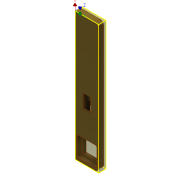
# Autodesk Inventor part: Hilla
Saved by Autodesk Inventor 2018 (Build 220112000, 112)
## iProperties
Created: 2019-09-21
Part Number: Hilla
Material: Lauan, Meranti
Document SubType Name: Modeling
Designer: ottar
Density: 0.416 g/cm^3
Appearance: Mahogany - Solid Stained Dark Medium Gloss
Author: ottar
Autodesk Inventor part; units mm, degrees
ref_plane "YZ Plane" through (0, 0, 0) normal (1, 0, 0) x (0, 1, 0)
ref_plane "XZ Plane" through (0, 0, 0) normal (0, 1, 0) x (-1, 0, 0)
sketch "Sketch1" plane through (0, 0, 0) normal (0, 1, 0) x (-1, 0, 0)
  line L0 (0, 0) -> (90, 0)
  line L1 (90, 0) -> (90, -500)
  line L2 (90, -500) -> (0, -500)
  line L3 (0, -500) -> (0, 0)
  dimension "d0" = 90
  dimension "d1" = 500
  constraints: 8 end point, 2 parallel, 1 horizontal, 1 perpendicular
  measures "d0" distance of L1.end L2.end
  measures "d1" distance of L0.end L1.end
extrude "Extrusion1" add sketch "Sketch1" along normal blind 25
sketch "Sketch6" plane through (0, 25, 0) normal (0, 1, 0) x (1, 0, 0)
  line L0 (-57.55, 311.9) -> (-32.45, 311.9)
  line L1 (-32.45, 311.9) -> (-32.45, 400)
  line L2 (-32.45, 400) -> (-57.55, 400)
  line L3 (-57.55, 400) -> (-57.55, 311.9)
  line L4 (-90, 500) -> (-90, 0) projected
  line L5 (0, 500) -> (-90, 500) projected
  point P0 (0, 0)
  dimension "d36" = 25.1
  dimension "d37" = 88.1
  dimension "d38" = 32.45
  dimension "d39" = 100
  constraints: 8 end point, 2 parallel, 1 horizontal, 1 perpendicular
  measures "d36" distance of L2.end L1.end
  measures "d37" distance of L0.end L1.end
  measures "d38" distance between parallel lines of L4 L3
  measures "d39" distance between parallel lines of L5 L2
extrude "Extrusion6" cut sketch "Sketch6" against normal blind 20
sketch "Sketch7" plane through (-32.45, 25, -311.9) normal (0, 0, -1) x (-1, 0, 0)
  line L0 (0, 0) -> (25.1, 0) projected
  line L1 (0, 0) -> (0, -20) projected
  line L2 (0, -20) -> (25.1, -20) projected
  line L3 (25.1, 0) -> (25.1, -20) projected
  line L4 (0, -4) -> (25.1, -4)
  line L5 (25.1, -4) -> (25.1, -23)
  line L6 (0, -4) -> (0, -23)
  line L7 (25.1, -23) -> (0, -23)
  point P0 (-32.45, -25)
  dimension "d42" = 16
  dimension "d43" = 19
  dimension "d44" = 19
  constraints: 8 end point, 2 vertical, 1 horizontal, 1 parallel, 1 point on line
  measures "d42" distance between parallel lines of L4 L2
  measures "d43" distance of L4.end L5.end
  measures "d44" distance of L4.start L6.end
ref_plane "Work Plane2" through (-32.45, 25, -313.9) normal (0, 0, -1) x (-1, 0, 0)
sketch "Sketch9" plane through (-32.45, 25, -313.9) normal (0, 0, -1) x (-1, 0, 0)
  line L0 (25.1, -4) -> (25.1, -23) projected
  line L1 (0, 0) -> (0, -20) projected
  line L2 (25.1, -23) -> (0, -23) projected
  line L3 (0, -23) -> (0, -4)
  line L4 (0, 0) -> (25.1, 0) projected
  line L5 (25.1, -4) -> (25.1, 0)
  line L6 (0, 0) -> (25.1, 0)
  line L7 (0, 0) -> (0, -4)
  line L8 (25.1, -3) -> (0, -3)
  point P0 (-32.45, -25)
  dimension "d97" = 3
  constraints: 10 end point, 2 point on line, 2 vertical, 1 collinear, 1 perpendicular
  measures "d97" distance between parallel lines of L4 L8
extrude "Extrusion9" cut sketch "Sketch9" against normal blind 22 contours L0 L2 L3 L1 L8 L5
sketch "Sketch12" plane through (0, 25, 0) normal (0, 1, 0) x (1, 0, 0)
  line L0 (-17.5, 480) -> (-72.5, 480)
  line L1 (-72.5, 480) -> (-72.5, 425)
  line L2 (-72.5, 425) -> (-17.5, 425)
  line L3 (-17.5, 425) -> (-17.5, 480)
  line L4 (0, 0) -> (0, 500) projected
  line L5 (-32.45, 311.9) -> (-57.55, 311.9) projected
  line L6 (0, 500) -> (-90, 500) projected
  dimension "d57" = 55
  dimension "d58" = 55
  dimension "d59" = 17.5
  dimension "d100" = 20
  constraints: 8 end point, 2 parallel, 1 horizontal, 1 perpendicular
  measures "d57" distance of L2.end L1.end
  measures "d58" distance of L1.end L0.end
  measures "d59" distance between parallel lines of L4 L3
  measures "d100" distance between parallel lines of L6 L0
extrude "Extrusion11" cut sketch "Sketch12" against normal blind 30
sketch "Sketch13" plane through (0, 0, 0) normal (0, -1, 0) x (1, 0, 0)
  line L0 (-72.5, -425) -> (-17.5, -425) projected
  line L1 (-17.5, -425) -> (-17.5, -480) projected
  line L2 (-17.5, -480) -> (-72.5, -480) projected
  line L3 (-72.5, -480) -> (-72.5, -425) projected
  line L4 (-7.5, -490) -> (-7.5, -415)
  line L5 (-7.5, -415) -> (-82.5, -415)
  line L6 (-82.5, -415) -> (-82.5, -490)
  line L7 (-82.5, -490) -> (-7.5, -490)
  point P0 (0, 0)
  dimension "d68" = 10
  constraints: 8 end point, 3 other
  measures "d68" distance between parallel lines of L4 L1
extrude "Extrusion12" cut sketch "Sketch13" against normal blind 14
sketch "Sketch14" plane through (0, 25, 0) normal (0, 1, 0) x (1, 0, 0)
  line L0 (-72.5, 425) -> (-72.5, 480) projected
  line L1 (-17.5, 425) -> (-72.5, 425) projected
  line L2 (-17.5, 480) -> (-17.5, 425) projected
  line L3 (-72.5, 480) -> (-17.5, 480) projected
  line L4 (-75, 482.5) -> (-75, 422.5) construction
  line L5 (-75, 422.5) -> (-15, 422.5) construction
  line L6 (-15, 422.5) -> (-15, 482.5) construction
  line L7 (-15, 482.5) -> (-75, 482.5) construction
  circle A0 centre (-75, 422.5) radius 2.05
  circle A1 centre (-75, 482.5) radius 2.05
  circle A2 centre (-15, 482.5) radius 2.05
  circle A3 centre (-15, 422.5) radius 2.05
  point P0 (0, 0)
  dimension "d69" = 2.5
  dimension "d70" = 4.1
  dimension "d71" = 4.1
  dimension "d72" = 4.1
  dimension "d73" = 4.1
  constraints: 8 end point, 4 centre point, 4 coincident, 3 other
  measures "d69" distance between parallel lines of L0 L4
  measures "d70" diameter of A0
  measures "d71" diameter of A1
  measures "d72" diameter of A2
  measures "d73" diameter of A3
fillet "Fillet14" radius 5 4 edges at (-82.5, 7, -415) (-7.5, 7, -415) (-7.5, 7, -490) (-82.5, 7, -490)
fillet "Fillet15" radius 2 8 edges at (-8.9645, 0, -488.5355) (-45, 0, -490) (-81.0355, 0, -488.5355) (-82.5, 0, -452.5) (-81.0355, 0, -416.4645) (-45, 0, -415) (-8.9645, 0, -416.4645) (-7.5, 0, -452.5)
sketch "Sketch15" plane through (0, 0, 0) normal (0, -1, 0) x (1, 0, 0)
  line L0 (-57.55, -311.625) -> (-32.45, -311.625)
  line L1 (-32.45, -311.625) -> (-32.45, -261.625)
  line L2 (-32.45, -261.625) -> (-57.55, -261.625)
  line L3 (-57.55, -261.625) -> (-57.55, -311.625)
  line L4 (-90, 0) -> (-90, -500) projected
  line L5 (-90, -500) -> (0, -500) projected
  point P0 (0, 0)
  dimension "d81" = 25.1
  dimension "d82" = 50
  dimension "d83" = 32.45
  dimension "d84" = 188.375
  constraints: 8 end point, 2 parallel, 1 horizontal, 1 perpendicular
  measures "d81" distance of L2.end L1.end
  measures "d82" distance of L1.end L0.end
  measures "d83" distance between parallel lines of L4 L3
  measures "d84" distance between parallel lines of L5 L0
extrude "Extrusion14" cut sketch "Sketch15" against normal blind 15
fillet "Fillet16" radius 2 1 edges at (-45, 15, -291.9)
fillet "Fillet17" radius 2 3 edges at (-32.45, 0, -286.625) (-57.55, 0, -286.625) (-45, 0, -311.625)
fillet "Fillet18" radius 5 3 edges at (0, 25, -250) (-45, 25, 0) (-45, 25, -500)
fillet "Fillet19" radius 15 4 edges at (-1.4645, 23.5355, -1.4645) (0, 10, 0) (-1.4645, 23.5355, -498.5355) (0, 10, -500)
sketch "Sketch22" plane through (-57.55, 2, -313.9) normal (0, 1, 0) x (1, 0, 0)
  line L0 (0, -2.275) -> (25.1, -2.275) projected
  line L1 (25.1, 0) -> (25.1, -2.275) projected
  line L2 (25.1, 0) -> (0, 0) projected
  line L3 (0, 0) -> (0, -2.275) projected
  point P0 (57.55, -313.9)
extrude "Extrusion18" cut sketch "Sketch22" against normal blind 6
sketch "Sketch23" plane through (0, 0, 0) normal (0, -1, 0) x (1, 0, 0)
  point P0 (0, 0)
sketch "Sketch24" plane through (0, 25, 0) normal (0, 1, 0) x (1, 0, 0)
  line L0 (-24.2952, 12.3012) -> (-24.2952, 52.9327) construction
  line L1 (-24.2952, 52.9327) -> (-73.6667, 52.9327) construction
  line L2 (-73.6667, 52.9327) -> (-73.6667, 12.3012) construction
  line L3 (-73.6667, 12.3012) -> (-24.2952, 12.3012) construction
  point P0 (0, 0)
  constraints: 2 other
extrude "Extrusion19" [suppressed]
sketch "Sketch25" plane through (0, 14, 0) normal (0, -1, 0) x (1, 0, 0)
  line L0 (-17.5, -480) -> (-17.5, -425) projected
  line L1 (-17.5, -425) -> (-72.5, -425) projected
  line L2 (-72.5, -480) -> (-17.5, -480) projected
  line L3 (-72.5, -425) -> (-72.5, -480) projected
  circle A0 centre (-75, -482.5) radius 2.05 projected
  circle A1 centre (-15, -482.5) radius 2.05 projected
  circle A2 centre (-15, -422.5) radius 2.05 projected
  circle A3 centre (-75, -422.5) radius 2.05 projected
  point P0 (0, 0)
extrude "Extrusion20" cut sketch "Sketch25" against normal blind 1 contours A0 | A1 | A2 | A3
body "Solid1"
